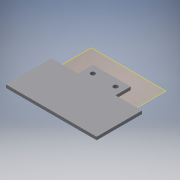
# Autodesk Inventor part: april_tag_2
Saved by Autodesk Inventor 2018 (Build 220112000, 112)
## iProperties
Created: 2018-06-13
Part Number: april_tag_2
Material: Generic
Document SubType Name: Modeling
Designer: bitbots
Density: 1 g/cm^3
Appearance: Default
Author: bitbots
Autodesk Inventor part; units mm, degrees
ref_plane "YZ Plane" through (0, 0, 0) normal (1, 0, 0) x (0, 1, 0)
ref_plane "XZ Plane" through (0, 0, 0) normal (0, 1, 0) x (-1, 0, 0)
ref_plane "XY Plane" through (0, 0, 0) normal (0, 0, 1) x (1, 0, 0)
ref_plane "Work Plane1" through (0, 0, 0) normal (0, 0, 1) x (1, 0, 0)
sketch "Sketch1" plane through (0, 0, 0) normal (0, 0, 1) x (1, 0, 0)
  circle A0 centre (15, -11) radius 1.5 projected
  circle A1 centre (30, -11) radius 1.5 projected
  line L0 (0, -20) -> (0, 4) construction
  line L1 (0, -20) -> (45, -20) construction
  line L2 (45, -20) -> (45, 4) construction
  line L3 (0, 4) -> (45, 4) construction
  line L4 (15, -11) -> (10, -11) construction
  line L5 (10, -11) -> (10, -6) construction
  line L6 (10, -6) -> (15, -6) construction
  line L7 (15, -6) -> (15, -11) construction
  line L8 (30, -11) -> (35, -11) construction
  line L9 (35, -11) -> (35, -6) construction
  line L10 (35, -6) -> (30, -6) construction
  line L11 (30, -6) -> (30, -11) construction
  line L12 (10, -6) -> (35, -6)
  line L13 (35, -6) -> (35, -16)
  line L14 (35, -16) -> (10, -16)
  line L15 (10, -16) -> (10, -6)
  line L16 (22.5, -16) -> (-7.5, -16)
  line L17 (-7.5, -16) -> (52.5, -16)
  line L18 (52.5, -16) -> (52.5, -46)
  line L19 (52.5, -46) -> (-7.5, -46)
  line L20 (-7.5, -46) -> (-7.5, -16)
  point P0 (0, 0)
  dimension "d0" = 5
  dimension "d1" = 5
  dimension "d2" = 5
  dimension "d3" = 5
  dimension "d4" = 10
  dimension "d5" = 30
  dimension "d6" = 60
  dimension "d7" = 30
  constraints: 34 end point, 8 parallel, 4 horizontal, 4 perpendicular, 1 midpoint, 1 point on line
  measures "d0" distance of L5.end L6.end
  measures "d1" distance of L4.end L5.end
  measures "d2" distance of L10.end L9.end
  measures "d3" distance of L9.end L8.end
  measures "d4" distance of L12.end L13.end
  measures "d5" distance of L16.start L16.end
  measures "d6" distance of L18.end L19.end
  measures "d7" distance of L17.end L18.end
extrude "Extrusion1" add sketch "Sketch1" along normal blind 2
body "Solid1"
